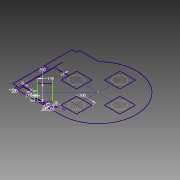
# Autodesk Inventor part: Foam_Right
Saved by Autodesk Inventor 2014 SP1 (Build 180222100, 222)
## iProperties
Created: 2014-01-13
Part Number: Foam_Right
Material: Generic
Document SubType Name: Modeling
Designer: tuleu
Density: 1 g/cm^3
Appearance: Default
Author: tuleu
Autodesk Inventor part; units mm, degrees
ref_plane "YZ Plane" through (0, 0, 0) normal (1, 0, 0) x (0, 1, 0)
ref_plane "XZ Plane" through (0, 0, 0) normal (0, 1, 0) x (-1, 0, 0)
ref_plane "XY Plane" through (0, 0, 0) normal (0, 0, 1) x (1, 0, 0)
sketch "Sketch1" plane through (0, 0, 0) normal (0, 1, 0) x (-1, 0, 0)
  line L0 (0, 490) -> (590, 490)
  line L1 (590, -350) -> (342.9286, -350)
  arc A0 (0, 490) -> (342.9286, -350) centre (0, 0) ccw
  line L2 (590, -310) -> (650, -310)
  line L3 (590, 450) -> (590, 490)
  line L4 (650, 450) -> (590, 450)
  line L5 (590, 90) -> (590, 50)
  line L6 (590, 90) -> (650, 90)
  line L7 (650, 450) -> (650, 90)
  line L8 (650, 50) -> (590, 50)
  line L9 (590, -310) -> (590, -350)
  line L10 (650, -310) -> (650, 50)
  circle A1 centre (280, 0) radius 75 construction
  circle A2 centre (0, 280) radius 75 construction
  circle A3 centre (-280, 0) radius 75 construction
  circle A4 centre (0, -280) radius 75 construction
  line L11 (0, 280) -> (0, -280) construction
  line L12 (280, 0) -> (-280, 0) construction
  line L13 (-100, 380) -> (-100, 180)
  line L14 (-100, 180) -> (100, 180)
  line L15 (100, 180) -> (100, 380)
  line L16 (380, 100) -> (180, 100)
  line L17 (180, 100) -> (180, -100)
  line L18 (180, -100) -> (380, -100)
  line L19 (-180, 100) -> (-380, 100)
  line L20 (-380, -100) -> (-180, -100)
  line L21 (-180, -100) -> (-180, 100)
  line L22 (100, -180) -> (-100, -180)
  line L23 (-100, -180) -> (-100, -380)
  line L24 (100, -380) -> (100, -180)
  line L25 (100, 280) -> (-100, 280) construction
  line L26 (280, 100) -> (280, -100) construction
  line L27 (435, 440) -> (525, 440) construction
  line L28 (550, 490) -> (550, 420)
  line L29 (550, 420) -> (298.4205, 420)
  line L30 (298.4205, 420) -> (248.4205, 470)
  line L31 (248.4205, 470) -> (148.6863, 470)
  line L32 (148.6863, 470) -> (96.6863, 418)
  line L33 (570, 490) -> (570, 412)
  line L34 (295.1068, 412) -> (245.1068, 462)
  line L35 (245.1068, 462) -> (152, 462)
  line L36 (152, 462) -> (100, 410)
  line L37 (100, 410) -> (1.5, 410)
  line L38 (100, 380) -> (100, 490) construction
  line L39 (570, 412) -> (570, -112.1213)
  line L40 (564, 409) -> (564, 1.5)
  line L41 (564, 1.5) -> (380, 1.5)
  line L42 (380, -1.5) -> (567, -1.5)
  line L43 (380, -100) -> (380, -1.5)
  line L44 (380, 1.5) -> (380, 100)
  line L45 (434.8707, 229.8097) -> (335.8757, 130.8148)
  line L46 (335.8757, 130.8148) -> (130.8148, 335.8757)
  line L47 (130.8148, 335.8757) -> (229.8097, 434.8707)
  line L48 (304.0559, 197.9899) -> (197.9899, 304.0559) construction
  line L49 (304.0559, 197.9899) -> (197.9899, 304.0559) construction
  arc A5 (261.6295, 367.6955) -> (197.9899, 304.0559) centre (229.8097, 335.8757) ccw construction
  line L50 (261.6295, 367.6955) -> (367.6955, 261.6295) construction
  arc A6 (304.0559, 197.9899) -> (367.6955, 261.6295) centre (335.8757, 229.8097) ccw construction
  line L51 (251.0229, 251.0229) -> (314.6625, 314.6625) construction
  line L52 (411.1213, 409) -> (333.4008, 331.2795)
  line L53 (409.8787, 412) -> (331.2795, 333.4008)
  line L54 (229.8097, 434.8707) -> (331.2795, 333.4008)
  line L55 (333.4008, 331.2795) -> (434.8707, 229.8097)
  line L56 (564, 409) -> (411.1213, 409)
  line L57 (409.8787, 412) -> (295.1068, 412)
  line L58 (-1.5, 410) -> (-1.5, 380)
  line L59 (1.5, 410) -> (1.5, 380)
  line L60 (-1.5, 410) -> (-100, 410)
  line L61 (-100, 380) -> (-100, 479.6874) construction
  line L62 (-380, 100) -> (-479.6874, 100) construction
  line L63 (-380, -100) -> (-479.6874, -100) construction
  line L64 (-100, -380) -> (-100, -479.6874) construction
  line L65 (100, 380) -> (1.5, 380)
  line L66 (-1.5, 380) -> (-100, 380)
  line L67 (96.6863, 418) -> (-1.5, 418)
  line L68 (-1.5, 418) -> (-1.5, 416)
  line L69 (-1.5, 416) -> (-102.4853, 416)
  line L70 (-410, 100) -> (-410, 1.5)
  line L71 (-410, 1.5) -> (-380, 1.5)
  line L72 (-380, -1.5) -> (-410, -1.5)
  line L73 (-410, -1.5) -> (-410, -100)
  line L74 (-380, 100) -> (-380, 1.5)
  line L75 (-380, -1.5) -> (-380, -100)
  line L76 (-100, 410) -> (-410, 100)
  line L77 (-102.4853, 416) -> (-416, 102.4853)
  line L78 (-416, 102.4853) -> (-416, -1.5)
  line L79 (-416, -1.5) -> (-413, -1.5)
  line L80 (-413, -1.5) -> (-413, -101.2426)
  line L81 (-100, -410) -> (-1.5, -410)
  line L82 (-1.5, -410) -> (-1.5, -380)
  line L83 (1.5, -380) -> (1.5, -413)
  line L84 (1.5, -413) -> (-101.2426, -413)
  line L85 (-100, -380) -> (-1.5, -380)
  line L86 (1.5, -380) -> (100, -380)
  line L87 (-410, -100) -> (-100, -410)
  line L88 (-101.2426, -413) -> (-413, -101.2426)
  line L89 (514.1421, -229.4975) -> (450.5025, -165.8579) construction
  arc A7 (485.8579, -130.5025) -> (450.5025, -165.8579) centre (468.1802, -148.1802) ccw construction
  line L90 (485.8579, -130.5025) -> (549.4975, -194.1421) construction
  arc A8 (514.1421, -229.4975) -> (549.4975, -194.1421) centre (531.8198, -211.8198) ccw construction
  line L91 (468.1802, -148.1802) -> (531.8198, -211.8198) construction
  line L92 (517.6777, -162.3223) -> (482.3223, -197.6777) construction
  line L93 (471.7157, -81.0051) -> (401.0051, -151.7157)
  line L94 (401.0051, -151.7157) -> (528.2843, -278.9949)
  line L95 (528.2843, -278.9949) -> (598.9949, -208.2843)
  line L96 (536.416, -145.7053) -> (570, -112.1213)
  line L97 (534.2947, -143.584) -> (567, -110.8787)
  line L98 (567, -110.8787) -> (567, -1.5)
  line L99 (598.9949, -208.2843) -> (536.416, -145.7053)
  line L100 (534.2947, -143.584) -> (471.7157, -81.0051)
  point P0 (0, 0)
  dimension "d1" = 200
  dimension "d3" = 20
  dimension "d4" = 8
  dimension "d5" = 8
  dimension "d6" = 135
  dimension "d8" = 8
  dimension "d9" = 20
  dimension "d11" = 20
  dimension "d12" = 20
  dimension "d13" = 6
  dimension "d14" = 3
  dimension "d15" = 290
  dimension "d17" = 25
  dimension "d19" = 3
  dimension "d20" = 140
  dimension "d21" = 30
  dimension "d22" = 8
  dimension "d23" = 11
  dimension "d24" = 3
  dimension "d25" = 30
  dimension "d26" = 8
  dimension "d27" = 6
  dimension "d29" = 30
  dimension "d30" = 3
  dimension "d31" = 6
  dimension "d32" = 6
  dimension "d33" = 3
  dimension "d34" = 30
  dimension "d35" = 3
  dimension "d36" = 3
  dimension "d37" = 3
  dimension "d39" = 180
  dimension "d40" = 3
  dimension "d41" = 3
  dimension "d42" = 100
  constraints: 190 end point, 50 parallel, 43 perpendicular, 10 collinear, 10 midpoint, 8 horizontal, 8 point on line, 6 point on circle, 2 vertical, 1 centre point, 26 other
  measures "d1" distance of L13.end L14.end
  measures "d3" distance between parallel lines of L0 L31
  measures "d4" distance between parallel lines of L35 L31
  measures "d5" distance between parallel lines of L32 L36
  measures "d6" angle of L32 L31
  measures "d8" distance between parallel lines of L30 L34
  measures "d9" distance between parallel lines of L29 L27
  measures "d11" distance between parallel lines of L33 L3
  measures "d12" distance between parallel lines of L28 L33
  measures "d13" distance between parallel lines of L39 L40
  measures "d14" distance between parallel lines of L41 L42
  measures "d15" distance between parallel lines of L45 L47
  measures "d17" distance between parallel lines of L46 L48
  measures "d19" distance between parallel lines of L52 L53
  measures "d20" distance between parallel lines of L46 L55
  measures "d21" distance between parallel lines of L54 L34
  measures "d22" distance between parallel lines of L57 L29
  measures "d23" distance between parallel lines of L56 L29
  measures "d24" distance between parallel lines of L58 L59
  measures "d25" distance between parallel lines of L65 L37
  measures "d26" distance between parallel lines of L37 L67
  measures "d27" distance between parallel lines of L60 L69
  measures "d29" distance between parallel lines of L70 L74
  measures "d30" distance between parallel lines of L72 L71
  measures "d31" distance between parallel lines of L76 L77
  measures "d32" distance between parallel lines of L78 L70
  measures "d33" distance between parallel lines of L73 L80
  measures "d34" distance between parallel lines of L81 L85
  measures "d35" distance between parallel lines of L82 L83
  measures "d36" distance between parallel lines of L81 L84
  measures "d37" distance between parallel lines of L88 L87
  measures "d39" distance between parallel lines of L95 L93
  measures "d40" distance between parallel lines of L96 L97
  measures "d41" distance between parallel lines of L98 L39
  measures "d42" distance between parallel lines of L94 L100
extrude "Extrusion1" add sketch "Sketch1" against normal blind 3 contours L0 L28 L29 L30 L31 L32 L67 L68 L69 L77 L78 L79 L80 L88 L84 L83 L86 L24 L22 L23 L85 L82 L81 L87 L73 L72 L75 L20 L21 L19 L74 L71 L70 L76 L60 L58 L66 L13 L14 L15 L65 L59 L37 L36 L35 L34 L57 L53 L54 L47 L46 L45 L55 L52 L56 L40 L41 L44 L16 L17 L18 L43 L42 L98 L97 L100 L93 L94 L95 L99 L96 L39 L33 L3 L4 L7 L6 L5 L8 L10 L2 L9 L1 A0
ref_plane "Work Plane1" through (0, -3, 0) normal (0, -1, 0) x (1, 0, 0)
sketch "Sketch2" plane through (0, -3, 0) normal (0, -1, 0) x (1, 0, 0)
  arc A0 (-342.9286, -350) -> (0, 490) centre (0, 0) ccw construction
  line L0 (0, 490) -> (-550, 490) construction
  line L1 (-550, 490) -> (-550, 420) construction
  line L2 (-550, 420) -> (-298.4205, 420) construction
  line L3 (-298.4205, 420) -> (-248.4205, 470) construction
  line L4 (-248.4205, 470) -> (-148.6863, 470) construction
  line L5 (-148.6863, 470) -> (-96.6863, 418) construction
  line L6 (-96.6863, 418) -> (1.5, 418) construction
  line L7 (1.5, 418) -> (1.5, 416) construction
  line L8 (1.5, 416) -> (102.4853, 416) construction
  line L9 (102.4853, 416) -> (416, 102.4853) construction
  line L10 (416, 102.4853) -> (416, -1.5) construction
  line L11 (416, -1.5) -> (413, -1.5) construction
  line L12 (413, -1.5) -> (413, -101.2426) construction
  line L13 (413, -101.2426) -> (101.2426, -413) construction
  line L14 (101.2426, -413) -> (-1.5, -413) construction
  line L15 (-1.5, -413) -> (-1.5, -380) construction
  line L16 (-1.5, -380) -> (-100, -380) construction
  line L17 (-100, -380) -> (-100, -180) construction
  line L18 (-100, -180) -> (100, -180) construction
  line L19 (100, -180) -> (100, -380) construction
  line L20 (100, -380) -> (1.5, -380) construction
  line L21 (1.5, -380) -> (1.5, -410) construction
  line L22 (1.5, -410) -> (100, -410) construction
  line L23 (100, -410) -> (410, -100) construction
  line L24 (410, -100) -> (410, -1.5) construction
  line L25 (410, -1.5) -> (380, -1.5) construction
  line L26 (380, -1.5) -> (380, -100) construction
  line L27 (380, -100) -> (180, -100) construction
  line L28 (180, -100) -> (180, 100) construction
  line L29 (180, 100) -> (380, 100) construction
  line L30 (380, 100) -> (380, 1.5) construction
  line L31 (380, 1.5) -> (410, 1.5) construction
  line L32 (410, 1.5) -> (410, 100) construction
  line L33 (410, 100) -> (100, 410) construction
  line L34 (100, 410) -> (1.5, 410) construction
  line L35 (1.5, 410) -> (1.5, 380) construction
  line L36 (1.5, 380) -> (100, 380) construction
  line L37 (100, 380) -> (100, 180) construction
  line L38 (100, 180) -> (-100, 180) construction
  line L39 (-100, 180) -> (-100, 380) construction
  line L40 (-100, 380) -> (-1.5, 380) construction
  line L41 (-1.5, 380) -> (-1.5, 410) construction
  line L42 (-1.5, 410) -> (-100, 410) construction
  line L43 (-100, 410) -> (-152, 462) construction
  line L44 (-152, 462) -> (-245.1068, 462) construction
  line L45 (-245.1068, 462) -> (-295.1068, 412) construction
  line L46 (-295.1068, 412) -> (-409.8787, 412) construction
  line L47 (-409.8787, 412) -> (-331.2795, 333.4008) construction
  line L48 (-331.2795, 333.4008) -> (-229.8097, 434.8707) construction
  line L49 (-229.8097, 434.8707) -> (-130.8148, 335.8757) construction
  line L50 (-130.8148, 335.8757) -> (-335.8757, 130.8148) construction
  line L51 (-335.8757, 130.8148) -> (-434.8707, 229.8097) construction
  line L52 (-434.8707, 229.8097) -> (-333.4008, 331.2795) construction
  line L53 (-333.4008, 331.2795) -> (-411.1213, 409) construction
  line L54 (-411.1213, 409) -> (-564, 409) construction
  line L55 (-564, 409) -> (-564, 1.5) construction
  line L56 (-564, 1.5) -> (-380, 1.5) construction
  line L57 (-380, 1.5) -> (-380, 100) construction
  line L58 (-380, 100) -> (-180, 100) construction
  line L59 (-180, 100) -> (-180, -100) construction
  line L60 (-180, -100) -> (-380, -100) construction
  line L61 (-380, -100) -> (-380, -1.5) construction
  line L62 (-380, -1.5) -> (-567, -1.5) construction
  line L63 (-567, -1.5) -> (-567, -110.8787) construction
  line L64 (-567, -110.8787) -> (-534.2947, -143.584) construction
  line L65 (-534.2947, -143.584) -> (-471.7157, -81.0051) construction
  line L66 (-471.7157, -81.0051) -> (-401.0051, -151.7157) construction
  line L67 (-401.0051, -151.7157) -> (-528.2843, -278.9949) construction
  line L68 (-528.2843, -278.9949) -> (-598.9949, -208.2843) construction
  line L69 (-598.9949, -208.2843) -> (-536.416, -145.7053) construction
  line L70 (-536.416, -145.7053) -> (-570, -112.1213) construction
  line L71 (-570, -112.1213) -> (-570, 490) construction
  line L72 (-570, 490) -> (-590, 490) construction
  line L73 (-590, 490) -> (-590, 450) construction
  line L74 (-590, 450) -> (-650, 450) construction
  line L75 (-650, 450) -> (-650, 90) construction
  line L76 (-650, 90) -> (-590, 90) construction
  line L77 (-590, 90) -> (-590, 50) construction
  line L78 (-590, 50) -> (-650, 50) construction
  line L79 (-650, 50) -> (-650, -310) construction
  line L80 (-650, -310) -> (-590, -310) construction
  line L81 (-590, -310) -> (-590, -350) construction
  line L82 (-590, -350) -> (-342.9286, -350) construction
  line L83 (-650, 450) -> (-590, 450)
  line L84 (-590, 490) -> (0, 490)
  line L85 (-590, 490) -> (-590, 450)
  line L86 (-650, 450) -> (-650, 90)
  line L87 (-650, 90) -> (-590, 90)
  line L88 (-590, 90) -> (-590, 50)
  line L89 (-590, 50) -> (-650, 50)
  line L90 (-650, -310) -> (-650, 50)
  line L91 (-650, -310) -> (-590, -310)
  line L92 (-590, -310) -> (-590, -350)
  line L93 (-590, -350) -> (-342.9286, -350)
  arc A1 (-342.9286, -350) -> (0, 490) centre (0, 0) ccw
  line L94 (-100, 380) -> (100, 380)
  line L95 (100, 380) -> (100, 180)
  line L96 (100, 180) -> (-100, 180)
  line L97 (-100, 180) -> (-100, 380)
  line L98 (180, 100) -> (380, 100)
  line L99 (380, 100) -> (380, -100)
  line L100 (380, -100) -> (180, -100)
  line L101 (180, -100) -> (180, 100)
  line L102 (-380, 100) -> (-180, 100)
  line L103 (-180, 100) -> (-180, -100)
  line L104 (-180, -100) -> (-380, -100)
  line L105 (-380, -100) -> (-380, 100)
  line L106 (-100, -180) -> (100, -180)
  line L107 (100, -180) -> (100, -380)
  line L108 (100, -380) -> (-100, -380)
  line L109 (-100, -380) -> (-100, -180)
  line L110 (-471.7157, -81.0051) -> (-401.0051, -151.7157)
  line L111 (-401.0051, -151.7157) -> (-528.2843, -278.9949)
  line L112 (-528.2843, -278.9949) -> (-598.9949, -208.2843)
  line L113 (-598.9949, -208.2843) -> (-471.7157, -81.0051)
  line L114 (-434.8707, 229.8097) -> (-229.8097, 434.8707)
  line L115 (-229.8097, 434.8707) -> (-130.8148, 335.8757)
  line L116 (-130.8148, 335.8757) -> (-335.8757, 130.8148)
  line L117 (-335.8757, 130.8148) -> (-434.8707, 229.8097)
  line L118 (-229.8097, 434.8707) -> (-130.8148, 335.8757) projected
  line L119 (-434.8707, 229.8097) -> (-333.4008, 331.2795) projected
  line L120 (-335.8757, 130.8148) -> (-434.8707, 229.8097) projected
  line L121 (-130.8148, 335.8757) -> (-335.8757, 130.8148) projected
  line L122 (-534.2947, -143.584) -> (-471.7157, -81.0051) projected
  line L123 (-471.7157, -81.0051) -> (-401.0051, -151.7157) projected
  line L124 (-401.0051, -151.7157) -> (-528.2843, -278.9949) projected
  line L125 (-528.2843, -278.9949) -> (-598.9949, -208.2843) projected
  point P0 (0, 0)
  constraints: 70 end point, 16 collinear, 13 parallel, 8 perpendicular, 4 horizontal, 2 point on circle, 1 centre point, 1 coincident, 1 tangent
extrude "Extrusion2" add sketch "Sketch2" along normal blind 3
body "Solid1"
